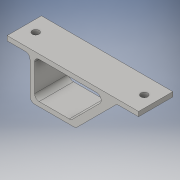
# Autodesk Inventor part: Motor_shroud
Saved by Autodesk Inventor 2016 (Build 200138000, 138)
## iProperties
Created: 2018-10-13
Part Number: Motor_shroud
Material: Generic
Document SubType Name: Modeling
Designer: Kyle
Density: 1 g/cm^3
Appearance: Default
Author: Kyle
Autodesk Inventor part; units mm, degrees
ref_plane "YZ Plane" through (0, 0, 0) normal (1, 0, 0) x (0, 1, 0)
ref_plane "XZ Plane" through (0, 0, 0) normal (0, 1, 0) x (-1, 0, 0)
ref_plane "XY Plane" through (0, 0, 0) normal (0, 0, 1) x (1, 0, 0)
sketch "Sketch1" plane through (0, 0, 0) normal (0, 0, 1) x (1, 0, 0)
  line L0 (0, -2) -> (0, -16)
  line L1 (2, -18) -> (19.1716, -18)
  line L2 (2, -2) -> (2, -14)
  line L3 (4, -16) -> (17.1716, -16)
  line L4 (20.5858, -17.4142) -> (37.4142, -0.5858)
  line L5 (18.5858, -15.4142) -> (30.5858, -3.4142)
  arc A0 (2, -14) -> (4, -16) centre (4, -14) ccw
  arc A1 (0, -16) -> (2, -18) centre (2, -16) ccw
  arc A2 (19.1716, -18) -> (20.5858, -17.4142) centre (19.1716, -16) ccw
  arc A3 (17.1716, -16) -> (18.5858, -15.4142) centre (17.1716, -14) ccw
  arc A4 (30.5858, -3.4142) -> (29.1716, 0) centre (29.1716, -2) ccw
  arc A5 (38.8284, 0) -> (37.4142, -0.5858) centre (38.8284, -2) ccw
  line L6 (2, -2) -> (2, -2)
  line L7 (-2, 0) -> (-10, 0)
  arc A6 (0, -2) -> (-2, 0) centre (-2, -2) ccw
  line L8 (-10, 0) -> (-10, 2)
  line L9 (-10, 2) -> (47.5, 2)
  line L10 (47.5, 2) -> (47.5, 0)
  arc A7 (4, 0) -> (2, -2) centre (4, -2) ccw
  line L11 (-10, 0) -> (-2, 0)
  line L12 (4, 0) -> (29.1716, 0)
  line L13 (38.8284, 0) -> (47.5, 0)
  line L14 (4, 0) -> (29.1716, 0)
  line L15 (38.8284, 0) -> (47.5, 0)
  line L16 (38.8284, 0) -> (38.8284, 2)
  point P0 (0, 0)
  point P1 (0, 0)
  point P2 (0, -18)
  point P3 (20, -18)
  point P4 (22, -16)
  point P5 (38, 0)
  point P6 (34, 0)
  point P7 (34, 0)
  dimension "d0" = 18
  dimension "d1" = 20
  dimension "d2" = 2
  dimension "d3" = 2
  dimension "d4" = 2
  dimension "d5" = 2
  dimension "d6" = 10
  dimension "d7" = 2
  dimension "d8" = 2
  dimension "d9" = 2
  constraints: 34 end point, 17 tangent, 16 point on circle, 12 point on line, 8 centre point, 8 perpendicular, 6 collinear, 4 horizontal, 3 equal radius, 2 vertical, 1 parallel, 2 other
  measures "d0" distance of point (0, 0) point (0, -18)
  measures "d1" distance of point (0, -18) point (20, -18)
  measures "d2" distance between parallel lines of L0 L2
  measures "d3" radius of A0
  measures "d4" radius of A4
  measures "d5" radius of A5
  measures "d6" distance of point (0, 0) L7.end
  measures "d7" radius of A6
  measures "d8" distance of L7.end L8.end
  measures "d9" radius of A7
extrude "Extrusion1" add sketch "Sketch1" along normal blind 15
sketch "Sketch2" plane through (38.8284, 0, 0) normal (0, -1, 0) x (1, 0, 0)
  line L0 (8.6716, 0) -> (-48.8284, 0) projected
  line L1 (-48.8284, 0) -> (-48.8284, 5)
  line L2 (-48.8284, 0) -> (-48.8284, 15) projected
  line L3 (-48.8284, 5) -> (-48.8284, 0)
  line L4 (8.6716, 15) -> (-48.8284, 15) projected
  line L5 (-48.8284, 0) -> (-48.8284, 15)
  line L6 (-48.8284, 15) -> (-48.8284, 7.5)
  line L7 (-48.8284, 0) -> (-48.8284, 15) projected
  line L8 (-40.8284, 15) -> (-38.8284, 15) projected
  line L9 (-48.8284, 15) -> (-38.8284, 15)
  line L10 (-38.8284, 15) -> (-43.8284, 15)
  line L11 (-43.8284, 15) -> (-43.8284, 7.5)
  line L12 (-48.8284, 15) -> (-40.8284, 15) projected
  circle A0 centre (-43.8284, 7.5) radius 1.5
  line L13 (-18.2426, 15) -> (-1.4142, 15) projected
  line L14 (8.6716, 15) -> (-1.4142, 15)
  line L15 (-1.4142, 15) -> (4.3358, 15)
  line L16 (0, 15) -> (8.6716, 15) projected
  line L17 (8.6716, 0) -> (8.6716, 15) projected
  line L18 (8.6716, 15) -> (-48.8284, 15)
  line L19 (-48.8284, 15) -> (-48.8284, 0)
  line L20 (-48.8284, 0) -> (8.6716, 0)
  line L21 (8.6716, 0) -> (8.6716, 15)
  line L22 (8.6716, 7.5) -> (3.6716, 7.5)
  circle A1 centre (3.6716, 7.5) radius 1.5
  line L23 (-43.8284, 7.5) -> (-48.8284, 7.5)
  point P0 (-38.8284, 0)
  dimension "d12" = 5
  dimension "d13" = 5
  dimension "d19" = 3
  dimension "d26" = 5
  dimension "d27" = 3
  constraints: 30 end point, 4 midpoint, 3 horizontal, 3 perpendicular, 2 centre point, 2 coincident, 2 collinear, 2 parallel, 1 point on line, 1 vertical
  measures "d12" distance of L0.end L1.end
  measures "d13" distance of L1.end L0.end
  measures "d19" diameter of A0
  measures "d26" distance of L22.start L22.end
  measures "d27" diameter of A1
extrude "Extrusion3" cut sketch "Sketch2" against normal blind 10 contours L23 L11 A0 | A0 L11 L23 | A1
body "Solid1"
